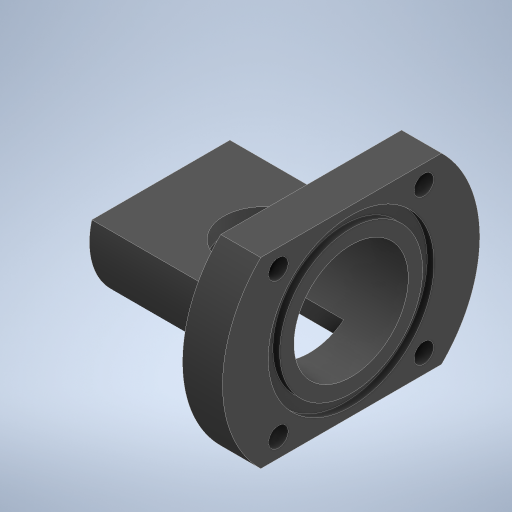
# Autodesk Inventor part: 022
Saved by Autodesk Inventor 2023 (Build 270158000, 158)
## iProperties
Created: 2021-11-20
Part Number: 022
Material: Aluminum 6061
Document SubType Name: Modeling
Designer: vinicius.miguel
Density: 2.7 g/cm^3
Appearance: Generic
Author: vinicius.miguel
Autodesk Inventor part; units mm, degrees
ref_plane "YZ Plane" through (0, 0, 0) normal (1, 0, 0) x (0, 1, 0)
ref_plane "XZ Plane" through (0, 0, 0) normal (0, 1, 0) x (-1, 0, 0)
ref_plane "XY Plane" through (0, 0, 0) normal (0, 0, 1) x (1, 0, 0)
sketch "Sketch4" plane through (0, 0, 0) normal (0, 0, 1) x (1, 0, 0)
  line L0 (0, 0) -> (7.3, 0)
  line L1 (7.3, 0) -> (7.3, 22.5)
  line L2 (7.3, 22.5) -> (0.3, 22.5)
  line L3 (0.3, 22.5) -> (0.3, 14)
  line L4 (0.3, 14) -> (1.5, 14)
  line L5 (1.5, 14) -> (1.5, 12.5)
  line L6 (1.5, 12.5) -> (0, 12.5)
  line L7 (0, 12.5) -> (0, 7.5)
  line L8 (0, 7.5) -> (0, 7.5)
  line L9 (0, 7.5) -> (0, 0)
  dimension "d44" = 25
  dimension "d45" = 1.5
  dimension "d46" = 1.2
  dimension "d47" = 1.5
  dimension "d53" = 45
  dimension "d58" = 7
  dimension "d59" = 15
  dimension "d60" = 0
  constraints: 20 end point, 8 perpendicular, 1 horizontal, 1 vertical
  measures "d44" diameter of L6 L0
  measures "d45" distance of L4.end L5.end
  measures "d46" distance between parallel lines of L5 L3
  measures "d47" distance of L5.end L6.end
  measures "d53" diameter of L2 L0
  measures "d58" distance of L1.end L2.end
  measures "d59" diameter of L8 L0
  measures "d60" distance of L7.end L8.end
revolve "Revolution2" add sketch "Sketch4" angle 360 about axis through (0, 0, 0) along (1, 0, 0)
sketch "Sketch7" plane through (7.3, 0, 0) normal (1, 0, 0) x (0, 0, -1)
  line L0 (-20, 26) -> (20, 26)
  line L1 (20, 26) -> (20, 16)
  line L2 (20, 16) -> (-20, 16)
  line L3 (-20, 16) -> (-20, 26)
  line L4 (20, -16) -> (-20, -16)
  line L5 (-20, -16) -> (-20, -26)
  line L6 (-20, -26) -> (20, -26)
  line L7 (20, -26) -> (20, -16)
  point P0 (0, 0)
  point P1 (0, 16)
  point P2 (0, -16)
  dimension "d61" = 16
  dimension "d62" = 16
  dimension "d63" = 10
  dimension "d64" = 10
  dimension "d65" = 20
  constraints: 16 end point, 4 parallel, 3 vertical alignment, 2 horizontal, 2 midpoint, 2 perpendicular
  measures "d61" distance from line of L2 point (0, 0)
  measures "d62" distance from line of point (0, 0) L4
  measures "d63" distance of L2.end L0.start
  measures "d64" distance of L4.end L5.end
  measures "d65" distance from line of L3 point (0, 0)
extrude "Extrusion2" cut sketch "Sketch7" against normal blind 20
sketch "Sketch10" plane through (0, 0, 0) normal (-1, 0, 0) x (0, 0, 1)
  circle A0 centre (0, 0) radius 12.5 projected
  circle A1 centre (0, 0) radius 12.5 projected
  line L0 (-12.5, 0) -> (12.5, 0) construction
  line L1 (-12.4984, 0.2) -> (12.4984, 0.2)
  line L2 (-12.0835, 3.2) -> (12.0835, 3.2)
  point P0 (-12.4984, 0.2)
  point P1 (12.4984, 0.2)
  dimension "d72" = 0.2
  dimension "d73" = 3
  constraints: 6 end point, 6 point on circle, 2 parallel, 1 coincident, 1 horizontal, 1 midpoint
  measures "d72" distance between parallel lines of L0 L1
  measures "d73" distance between parallel lines of L1 L2
extrude "Extrusion4" add sketch "Sketch10" along normal blind 26 contours L1 A0 L2
sketch "Sketch11" plane through (0, 3.2, 12.0835) normal (0, 1, 0) x (1, 0, 0)
  circle A0 centre (-8, 12.0835) radius 5 construction
  circle A1 centre (-8, 12.0835) radius 7
  point P0 (0, 12.0835)
  dimension "d76" = 14
  constraints: 1 centre point, 1 coincident
  measures "d76" diameter of A1
extrude "Extrusion5" cut sketch "Sketch11" against normal through all
sketch "Sketch12" plane through (0, 0, 0) normal (-1, 0, 0) x (0, 0, 1)
  line L0 (12.4984, 0.2) -> (-12.4984, 0.2) projected
  arc A0 (-12.4984, 0.2) -> (12.4984, 0.2) centre (0, 0) ccw projected
  line L1 (-6, 0.2) -> (-6, -10.9659)
  circle A1 centre (0, 0) radius 12.5 projected
  line L2 (12.4984, 0.2) -> (-12.4984, 0.2) projected
  line L3 (6, 0.2) -> (6, -10.9659)
  line L4 (-12.4984, 0.2) -> (12.4984, 0.2) projected
  dimension "d79" = 6
  dimension "d80" = 6
  constraints: 4 end point, 3 perpendicular, 2 point on circle, 2 point on line, 1 vertical
  measures "d79" distance from line of L3 point (0, 0)
  measures "d80" distance from line of L1 point (0, 0)
extrude "Extrusion6" add sketch "Sketch12" along normal blind 26 contours A0 L3 L0 | L0 L1 A0
sketch "Sketch13" plane through (7.3, 0, 0) normal (1, 0, 0) x (0, 0, -1)
  circle A0 centre (0, 0) radius 12.5 projected
  circle A1 centre (0, 0) radius 10
  dimension "d83" = 20
  constraints: 1 centre point, 1 coincident
  measures "d83" diameter of A1
extrude "Extrusion7" cut sketch "Sketch13" against normal blind 15 contours A1
sketch "Sketch14" plane through (7.3, 0, 0) normal (1, 0, 0) x (0, 0, -1)
  circle A0 centre (0, 0) radius 12.5 projected
  circle A1 centre (0, 0) radius 14.5
  dimension "d86" = 2
  constraints: 1 centre point
  measures "d86" radial gap between concentric circles of A0 A1
extrude "Extrusion8" cut sketch "Sketch14" against normal blind 1.2
sketch "Sketch15" plane through (7.3, 0, 0) normal (1, 0, 0) x (0, 0, -1)
  line L0 (0, 0) -> (12.7279, -12.7279)
  line L1 (0, 0) -> (18, 0) construction
  dimension "d89" = 18
  dimension "d90" = 45
  constraints: 4 end point, 1 coincident, 1 equal length, 1 horizontal
  measures "d89" distance of L0.start L0.end
  measures "d90" angle of L0 L1
hole "Hole3" at (7.3, -12.7279, -12.7279) direction (-1, 0, 0) diameter 3.4 end through all clearance for "Flat Head Machine Screw" size "M3" standard "Ansi Metric M Profile"
pattern_circular "Circular Pattern2" count 4 over 360 about axis through (0.75, 0, 0) along (1, 0, 0) of "Hole3"
equation "\"d62\" = d61"
equation "\"d64\" = d63"
equation "\"d80\" = d79"
body "Solid2"
